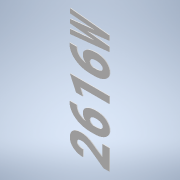
# Autodesk Inventor part: Licence plate numbers
Saved by Autodesk Inventor 2022 (Build 260153070, 153G)
## iProperties
Created: 2021-09-06
Part Number: Licence plate numbers
Material: Generic
Document SubType Name: Modeling
Designer: Main Account
Density: 1 g/cm^3
Appearance: Default
Author: Main Account
Autodesk Inventor part; units mm, degrees
ref_plane "YZ Plane" through (0, 0, 0) normal (1, 0, 0) x (0, 1, 0)
ref_plane "XZ Plane" through (0, 0, 0) normal (0, 1, 0) x (-1, 0, 0)
ref_plane "XY Plane" through (0, 0, 0) normal (0, 0, 1) x (1, 0, 0)
sketch "Sketch1" plane through (0, 0, 0) normal (0, 0, 1) x (1, 0, 0)
  line L0 (-16, -36.75) -> (-16, -53.25) construction
  line L1 (-16, -53.25) -> (16, -53.25) construction
  line L2 (16, -53.25) -> (16, -36.75) construction
  line L3 (16, -36.75) -> (-16, -36.75) construction
  line L4 (-16, -18.75) -> (-16, -35.25) construction
  line L5 (-16, -35.25) -> (16, -35.25) construction
  line L6 (16, -35.25) -> (16, -18.75) construction
  line L7 (16, -18.75) -> (-16, -18.75) construction
  line L8 (-16, -0.75) -> (-16, -17.25) construction
  line L9 (-16, -17.25) -> (16, -17.25) construction
  line L10 (16, -17.25) -> (16, -0.75) construction
  line L11 (16, -0.75) -> (-16, -0.75) construction
  line L12 (-16, 17.25) -> (-16, 0.75) construction
  line L13 (-16, 0.75) -> (16, 0.75) construction
  line L14 (16, 0.75) -> (16, 17.25) construction
  line L15 (16, 17.25) -> (-16, 17.25) construction
  line L16 (-16, 35.25) -> (-16, 18.75) construction
  line L17 (-16, 18.75) -> (16, 18.75) construction
  line L18 (16, 18.75) -> (16, 35.25) construction
  line L19 (16, 35.25) -> (-16, 35.25) construction
  line L20 (-16, -35.25) -> (-16, -18.75) construction
  line L21 (-16, -18.75) -> (16, -18.75) construction
  line L22 (16, -18.75) -> (16, -35.25) construction
  line L23 (16, -35.25) -> (-16, -35.25) construction
  line L24 (-16, -17.25) -> (-16, -0.75) construction
  line L25 (-16, -0.75) -> (16, -0.75) construction
  line L26 (16, -0.75) -> (16, -17.25) construction
  line L27 (16, -17.25) -> (-16, -17.25) construction
  line L28 (-16, -53.25) -> (-16, -36.75) construction
  line L29 (-16, -36.75) -> (16, -36.75) construction
  line L30 (16, -36.75) -> (16, -53.25) construction
  line L31 (16, -53.25) -> (-16, -53.25) construction
  line L32 (16, 0.75) -> (-16, 0.75) construction
  line L33 (-16, 0.75) -> (-16, 17.25) construction
  line L34 (-16, 17.25) -> (16, 17.25) construction
  line L35 (16, 17.25) -> (16, 0.75) construction
  line L36 (16, 18.75) -> (-16, 18.75) construction
  line L37 (-16, 18.75) -> (-16, 35.25) construction
  line L38 (-16, 35.25) -> (16, 35.25) construction
  line L39 (16, 35.25) -> (16, 18.75) construction
  line L40 (14.1658, -37.6407) -> (14.1658, -52.2441)
  line L41 (14.1658, -52.2441) -> (9.9276, -52.2441)
  line L42 (9.9276, -52.2441) -> (0.5067, -45.5183)
  spline S0 degree 2 poles (0.5067, -45.5183) (-3.2708, -43.0306) (-5.482, -43.0306) knots 0 0 0 1 1 1
  spline S1 degree 2 poles (-5.482, -43.0306) (-7.2787, -43.0306) (-9.1675, -44.2053) (-9.1675, -45.334) knots 0 0 0 1 2 2 2
  spline S2 degree 2 poles (-9.1675, -45.334) (-9.1675, -46.4396) (-6.6568, -47.8216) (-4.791, -47.8216) knots 0 0 0 1 2 2 2
  line L43 (-4.791, -47.8216) -> (-4.791, -52.6818)
  spline S3 degree 2 poles (-4.791, -52.6818) (-7.3478, -52.6818) (-11.7012, -50.7469) (-14.1658, -47.3379) (-14.1658, -45.2188) knots 0 0 0 1 2 3 3 3
  spline S4 degree 2 poles (-14.1658, -45.2188) (-14.1658, -41.8098) (-9.9736, -38.1474) (-6.0809, -38.1474) knots 0 0 0 1 2 2 2
  spline S5 degree 2 poles (-6.0809, -38.1474) (-4.4225, -38.1474) (-1.2899, -39.0688) (2.1421, -41.0267) (4.9983, -43.1688) knots 0 0 0 1 2 3 3 3
  line L44 (4.9983, -43.1688) -> (9.1675, -45.8868)
  line L45 (9.1675, -45.8868) -> (9.1675, -37.6407)
  line L46 (9.1675, -37.6407) -> (14.1658, -37.6407)
  line L47 (-14.3616, -22.543) -> (-9.2711, -22.543)
  line L48 (-9.2711, -22.543) -> (-9.2711, -22.7503)
  spline S6 degree 2 poles (-9.2711, -22.7503) (-9.2711, -25.4683) (-5.816, -28.9694) (-2.7295, -29.384) knots 0 0 0 1 2 2 2
  spline S7 degree 2 poles (-2.7295, -29.384) (-4.8716, -27.7256) (-4.8716, -25.2379) knots 0 0 0 1 1 1
  spline S8 degree 2 poles (-4.8716, -25.2379) (-4.8716, -22.5199) (0.4261, -19.2952) (4.7334, -19.2952) knots 0 0 0 1 2 2 2
  spline S9 degree 2 poles (4.7334, -19.2952) (7.3823, -19.2952) (11.8509, -21.184) (14.3616, -24.5469) (14.3616, -26.6199) knots 0 0 0 1 2 3 3 3
  spline S10 degree 2 poles (14.3616, -26.6199) (14.3616, -28.8312) (11.6666, -32.3554) (6.6222, -34.3132) (3.3514, -34.3363) knots 0 0 0 1 2 3 3 3
  line L49 (3.3514, -34.3363) -> (0.7486, -34.3363)
  spline S11 degree 2 poles (0.7486, -34.3363) (-3.5587, -34.3363) (-10.4458, -31.5492) (-14.3616, -26.4126) (-14.3616, -23.28) knots 0 0 0 1 2 3 3 3
  line L50 (-14.3616, -23.28) -> (-14.3616, -22.543)
  spline S12 degree 2 poles (0.0806, -26.9194) (0.0806, -27.8868) (1.2784, -29.1767) (2.1306, -29.4992) knots 0 0 0 1 2 2 2
  line L51 (2.1306, -29.4992) -> (4.0655, -29.4992)
  spline S13 degree 2 poles (4.0655, -29.4992) (9.3632, -29.4992) (9.3632, -26.7351) knots 0 0 0 1 1 1
  spline S14 degree 2 poles (9.3632, -26.7351) (9.3632, -25.6295) (6.7144, -24.1553) (4.7104, -24.1553) knots 0 0 0 1 2 2 2
  spline S15 degree 2 poles (4.7104, -24.1553) (2.6604, -24.1553) (0.0806, -25.6525) (0.0806, -26.9194) knots 0 0 0 1 2 2 2
  line L52 (13.97, -5.5104) -> (13.97, -10.3705)
  line L53 (13.97, -10.3705) -> (-6.6913, -10.3705)
  line L54 (-6.6913, -10.3705) -> (-4.8256, -15.1385)
  line L55 (-4.8256, -15.1385) -> (-9.7318, -15.1385)
  line L56 (-9.7318, -15.1385) -> (-13.97, -5.948)
  line L57 (-13.97, -5.948) -> (-13.97, -5.5104)
  line L58 (-13.97, -5.5104) -> (13.97, -5.5104)
  line L59 (-14.3616, 13.457) -> (-9.2711, 13.457)
  line L60 (-9.2711, 13.457) -> (-9.2711, 13.2497)
  spline S16 degree 2 poles (-9.2711, 13.2497) (-9.2711, 10.5317) (-5.816, 7.0306) (-2.7295, 6.616) knots 0 0 0 1 2 2 2
  spline S17 degree 2 poles (-2.7295, 6.616) (-4.8716, 8.2744) (-4.8716, 10.7621) knots 0 0 0 1 1 1
  spline S18 degree 2 poles (-4.8716, 10.7621) (-4.8716, 13.4801) (0.4261, 16.7048) (4.7334, 16.7048) knots 0 0 0 1 2 2 2
  spline S19 degree 2 poles (4.7334, 16.7048) (7.3823, 16.7048) (11.8509, 14.816) (14.3616, 11.4531) (14.3616, 9.3801) knots 0 0 0 1 2 3 3 3
  spline S20 degree 2 poles (14.3616, 9.3801) (14.3616, 7.1688) (11.6666, 3.6446) (6.6222, 1.6868) (3.3514, 1.6637) knots 0 0 0 1 2 3 3 3
  line L61 (3.3514, 1.6637) -> (0.7486, 1.6637)
  spline S21 degree 2 poles (0.7486, 1.6637) (-3.5587, 1.6637) (-10.4458, 4.4508) (-14.3616, 9.5874) (-14.3616, 12.72) knots 0 0 0 1 2 3 3 3
  line L62 (-14.3616, 12.72) -> (-14.3616, 13.457)
  spline S22 degree 2 poles (0.0806, 9.0806) (0.0806, 8.1132) (1.2784, 6.8233) (2.1306, 6.5008) knots 0 0 0 1 2 2 2
  line L63 (2.1306, 6.5008) -> (4.0655, 6.5008)
  spline S23 degree 2 poles (4.0655, 6.5008) (9.3632, 6.5008) (9.3632, 9.2649) knots 0 0 0 1 1 1
  spline S24 degree 2 poles (9.3632, 9.2649) (9.3632, 10.3705) (6.7144, 11.8447) (4.7104, 11.8447) knots 0 0 0 1 2 2 2
  spline S25 degree 2 poles (4.7104, 11.8447) (2.6604, 11.8447) (0.0806, 10.3475) (0.0806, 9.0806) knots 0 0 0 1 2 2 2
  line L64 (3.5587, 30.2247) -> (-13.97, 31.768)
  line L65 (-13.97, 31.768) -> (-13.97, 34.9927)
  line L66 (-13.97, 34.9927) -> (13.97, 32.1365)
  line L67 (13.97, 32.1365) -> (13.97, 28.7506)
  line L68 (13.97, 28.7506) -> (-1.9464, 26.9539)
  line L69 (-1.9464, 26.9539) -> (13.97, 25.1803)
  line L70 (13.97, 25.1803) -> (13.97, 21.8174)
  line L71 (13.97, 21.8174) -> (-13.97, 18.9382)
  line L72 (-13.97, 18.9382) -> (-13.97, 22.1859)
  line L73 (-13.97, 22.1859) -> (3.5587, 23.7292)
  line L74 (3.5587, 23.7292) -> (-13.97, 25.5719)
  line L75 (-13.97, 25.5719) -> (-13.97, 28.336)
  line L76 (-13.97, 28.336) -> (3.5587, 30.2247)
  point P0 (0, 0)
  constraints: 10 coincident, 10 other
extrude "Extrusion1" add sketch "Sketch1" along normal blind 0.508
body "Solid1"
